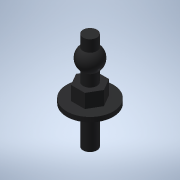
# Autodesk Inventor part: front_plate_screw
Saved by Autodesk Inventor 2020 (Build 240168000, 168)
## iProperties
Created: 2016-01-01
Part Number: front_plate_screw
Material: Genérico
Document SubType Name: Modeling
Designer: MIGUEL ANGEL
Density: 1 g/cm^3
Appearance: Goma - Negro
Author: MIGUEL ANGEL
Autodesk Inventor part; units mm, degrees
ref_plane "YZ Plane" through (0, 0, 0) normal (1, 0, 0) x (0, 1, 0)
ref_plane "XZ Plane" through (0, 0, 0) normal (0, 1, 0) x (-1, 0, 0)
ref_plane "XY Plane" through (0, 0, 0) normal (0, 0, 1) x (1, 0, 0)
sketch "Boceto1" plane through (0, 0, 0) normal (0, 0, 1) x (1, 0, 0)
  circle A0 centre (0, 0) radius 3
  dimension "d0" = 6
  constraints: 1 centre point, 1 coincident
  measures "d0" diameter of A0
extrude "Extrusión1" add sketch "Boceto1" along normal blind 16
sketch "Boceto2" plane through (0, 0, 16) normal (0, 0, 1) x (1, 0, 0)
  circle A0 centre (0, 0) radius 10
  dimension "d3" = 20
  constraints: 1 centre point, 1 coincident
  measures "d3" diameter of A0
extrude "Extrusión2" add sketch "Boceto2" along normal blind 2
sketch "Boceto3" plane through (0, 0, 18) normal (0, 0, 1) x (1, 0, 0)
  circle A0 centre (0, 0) radius 3 projected
  line L0 (6, 0) -> (3, -5.1962)
  line L1 (3, -5.1962) -> (-3, -5.1962)
  line L2 (-3, -5.1962) -> (-6, 0)
  line L3 (-6, 0) -> (-3, 5.1962)
  line L4 (-3, 5.1962) -> (3, 5.1962)
  line L5 (3, 5.1962) -> (6, 0)
  dimension "d6" = 6
  constraints: 12 end point, 1 coincident, 13 other
  measures "d6" distance of L3.end L4.end
extrude "Extrusión3" add sketch "Boceto3" along normal blind 6 contours A0 | L0 L1 L2 L3 L4 L5
sketch "Boceto4" plane through (0, 0, 24) normal (0, 0, 1) x (1, 0, 0)
  circle A0 centre (0, 0) radius 3
  dimension "d9" = 6
  constraints: 1 centre point, 1 coincident
  measures "d9" diameter of A0
extrude "Extrusión4" add sketch "Boceto4" along normal blind 18
sketch "Boceto5" plane through (0, 0, 0) normal (1, 0, 0) x (0, 1, 0)
  line L0 (3, 42) -> (-3, 42) projected
  line L1 (-3, 24) -> (3, 24) projected
  arc A0 (0, 28) -> (0, 38) centre (0, 33) ccw
  line L2 (3, 24) -> (3, 42) projected
  line L3 (-3, 24) -> (-3, 42) projected
  line L4 (0, 43.0217) -> (0, 25.7964)
  point P0 (0, 0)
  point P1 (3, 33)
  point P2 (0, 24)
  dimension "d12" = 10
  constraints: 2 end point, 2 midpoint, 2 point on circle, 2 point on line, 1 centre point, 1 horizontal alignment, 1 vertical, 1 vertical alignment
  measures "d12" diameter of A0
revolve "Revolución1" add sketch "Boceto5" angle 360 about axis through (0, 0, 43.0217) along (0, 0, -1) contours L2 A0 L4 | A0 L2
